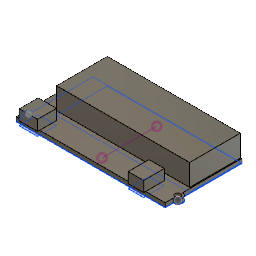
Dashboard Modell (Autodesk Fusion 360 design; units mm, degrees)
Autodesk Fusion 360 part; units mm, degrees
sketch "Skizze1" plane through (0, 0, 0) normal (0, 1, 0) x (1, 0, 0)
  line L0 (-28.3, 2.34) -> (28.3, 2.34)
  line L1 (28.3, -26.86) -> (-28.3, -26.86)
  line L2 (0, -1.75) -> (0, -22.5)
  circle A0 centre (28.3, -22.03) radius 1.1
  circle A1 centre (-28.3, -22.03) radius 1.1
  line L3 (-22.6, 2.09) -> (27.9, 2.09)
  line L4 (27.9, 2.09) -> (27.9, -17.21)
  line L5 (27.9, -17.21) -> (-22.6, -17.21)
  line L6 (-22.6, -17.21) -> (-22.6, 2.09)
  line L7 (-28.3, -20.23) -> (-28.3, 2.34)
  line L8 (28.3, 2.34) -> (28.3, -20.23)
  line L9 (28.3, -23.83) -> (28.3, -26.86)
  arc A2 (28.3, -23.83) -> (28.3, -20.23) centre (28.3, -22.03) ccw
  arc A3 (-28.3, -20.23) -> (-28.3, -23.83) centre (-28.3, -22.03) ccw
  line L10 (-28.3, -26.86) -> (-28.3, -23.83)
  line L11 (-19.3, -27.66) -> (-26.3, -27.66)
  line L12 (-26.3, -27.66) -> (-26.3, -20.46)
  line L13 (-26.3, -20.46) -> (-19.3, -20.46)
  line L14 (-19.3, -20.46) -> (-19.3, -27.66)
  line L15 (15.05, -19.75) -> (20.9, -19.75)
  line L16 (20.9, -19.75) -> (20.9, -27.62)
  line L17 (20.9, -27.62) -> (15.05, -27.62)
  line L18 (15.05, -27.62) -> (15.05, -19.75)
  dimension "d3" = 29.2
  dimension "d4" = 56.6
  dimension "d5" = 4.83
  dimension "d6" = 3.6
  dimension "d7" = 2.2
  dimension "d8" = 5.7
  dimension "d9" = 50.5
  dimension "d10" = 19.3
  dimension "d11" = 0.25
  dimension "d17" = 2
  dimension "d19" = 0.8
  dimension "d20" = 6.4
  dimension "d21" = 7
  dimension "d22" = 7.4
  dimension "d23" = 5.85
  dimension "d24" = 0.76
  dimension "d25" = 7.11
  measures "d3" distance of origin
  measures "d6" diameter of A2
  measures "d7" diameter of A0
  measures "d8" distance of L6 L10
  measures "d11" distance of L0 L3
  measures "d17" distance of L10 L12
  measures "d19" distance of L1 L11
  measures "d20" distance of L1 L13
  measures "d21" distance of L12 L14
  measures "d22" distance of L9 L16
  measures "d23" distance of origin
  measures "d24" distance of L1 L17
  measures "d25" distance of L1 L15
extrude "Extrusion1" add sketch "Skizze1" along normal blind 1.6 contours L0 L1 L7 L8 L9 A2 A3 L10 L12 L13 L14 L15 L16 L18 | L1 L12 L13 L14 | L1 L15 L16 L18 | L3 L4 L5 L6
extrude "Extrusion2" add sketch "Skizze1" along normal blind 8.2 from surface at 1.6 contours L3 L4 L5 L6
extrude "Extrusion3" add sketch "Skizze1" along normal blind 4 from surface at 1.6 contours L1 L12 L13 L14 | L1 L11 L12 L14 | L1 L16 L17 L18 | L1 L15 L16 L18
